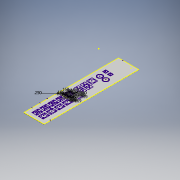
# Autodesk Inventor part: Box Connector Panel
Saved by Autodesk Inventor 2017 (Build 210142000, 142)
## iProperties
Created: 2017-03-01
Part Number: Box Connector Panel
Material: Generic
Document SubType Name: Modeling
Designer: slukej
Density: 1 g/cm^3
Appearance: Default
Author: slukej
Autodesk Inventor part; units mm, degrees
ref_plane "YZ Plane" through (0, 0, 0) normal (1, 0, 0) x (0, 1, 0)
ref_plane "XZ Plane" through (0, 0, 0) normal (0, 1, 0) x (-1, 0, 0)
ref_plane "XY Plane" through (0, 0, 0) normal (0, 0, 1) x (1, 0, 0)
sketch "Connector Plate" plane through (0, 0, 0) normal (0, 1, 0) x (-1, 0, 0)
  line L0 (-113.7687, 596.4285) -> (-243.9437, 596.4285)
  line L1 (-243.9437, 596.4285) -> (-243.9437, -13.1715)
  line L2 (-243.9437, -13.1715) -> (-113.7687, -13.1715)
  line L3 (-113.7687, -13.1715) -> (-113.7687, 596.4285)
  point P0 (0, 0)
  dimension "d0" = 130.175
  dimension "d1" = 609.6
  constraints: 8 end point, 2 parallel, 1 horizontal, 1 perpendicular
  measures "d0" distance of L2.end L1.end
  measures "d1" distance of L0.end L1.end
extrude "Extrusion1" add sketch "Connector Plate" along normal blind 3.175
sketch "DT04-2P - Exterior Panel (LS)" plane through (0, 3.175, 0) normal (0, 1, 0) x (1, 0, 0)
  line L0 (150.9797, -559.9795) -> (159.1077, -559.9795)
  line L1 (164.1877, -554.8995) -> (164.1877, -546.6445)
  line L2 (159.1077, -541.5645) -> (150.9797, -541.5645)
  line L3 (145.8997, -546.6445) -> (145.8997, -554.8995)
  circle A0 centre (143.8169, -565.9485) radius 2.159
  arc A1 (145.8997, -554.8995) -> (150.9797, -559.9795) centre (150.9797, -554.8995) ccw
  arc A2 (159.1077, -559.9795) -> (164.1877, -554.8995) centre (159.1077, -554.8995) ccw
  arc A3 (150.9797, -541.5645) -> (145.8997, -546.6445) centre (150.9797, -546.6445) ccw
  arc A4 (164.1877, -546.6445) -> (159.1077, -541.5645) centre (159.1077, -546.6445) ccw
  circle A5 centre (166.2705, -565.9485) radius 2.159
  circle A6 centre (143.8169, -535.5955) radius 2.159
  circle A7 centre (166.2705, -535.5955) radius 2.159
  line L4 (139.1687, -571.0285) -> (170.9187, -571.0285)
  line L5 (170.9187, -571.0285) -> (170.9187, -530.5155)
  line L6 (170.9187, -530.5155) -> (139.1687, -530.5155)
  line L7 (139.1687, -530.5155) -> (139.1687, -571.0285)
  line L8 (113.7687, -596.4285) -> (243.9437, -596.4285) projected
  line L9 (243.9437, -596.4285) -> (243.9437, 13.1715) projected
  line L10 (243.9437, 13.1715) -> (113.7687, 13.1715) projected
  line L11 (113.7687, 13.1715) -> (113.7687, -596.4285) projected
  line L12 (113.7687, 13.1715) -> (113.7687, -596.4285) projected
  line L13 (113.7687, -596.4285) -> (243.9437, -596.4285) projected
  line L14 (243.9437, 13.1715) -> (113.7687, 13.1715) projected
  arc A8 (150.9797, -490.7645) -> (145.8997, -495.8445) centre (150.9797, -495.8445) ccw
  line L15 (159.1077, -490.7645) -> (150.9797, -490.7645)
  arc A9 (164.1877, -495.8445) -> (159.1077, -490.7645) centre (159.1077, -495.8445) ccw
  arc A10 (145.8997, -504.0995) -> (150.9797, -509.1795) centre (150.9797, -504.0995) ccw
  line L16 (139.1687, -479.7155) -> (139.1687, -520.2285)
  arc A11 (159.1077, -509.1795) -> (164.1877, -504.0995) centre (159.1077, -504.0995) ccw
  line L17 (170.9187, -520.2285) -> (170.9187, -479.7155)
  line L18 (170.9187, -479.7155) -> (139.1687, -479.7155)
  circle A12 centre (166.2705, -484.7955) radius 2.159
  circle A13 centre (166.2705, -515.1485) radius 2.159
  line L19 (150.9797, -509.1795) -> (159.1077, -509.1795)
  circle A14 centre (143.8169, -515.1485) radius 2.159
  line L20 (164.1877, -504.0995) -> (164.1877, -495.8445)
  line L21 (145.8997, -495.8445) -> (145.8997, -504.0995)
  circle A15 centre (143.8169, -484.7955) radius 2.159
  line L22 (139.1687, -520.2285) -> (170.9187, -520.2285)
  arc A16 (150.9797, -439.9645) -> (145.8997, -445.0445) centre (150.9797, -445.0445) ccw
  line L23 (159.1077, -439.9645) -> (150.9797, -439.9645)
  arc A17 (164.1877, -445.0445) -> (159.1077, -439.9645) centre (159.1077, -445.0445) ccw
  arc A18 (145.8997, -453.2995) -> (150.9797, -458.3795) centre (150.9797, -453.2995) ccw
  line L24 (139.1687, -428.9155) -> (139.1687, -469.4285)
  arc A19 (159.1077, -458.3795) -> (164.1877, -453.2995) centre (159.1077, -453.2995) ccw
  line L25 (170.9187, -469.4285) -> (170.9187, -428.9155)
  line L26 (170.9187, -428.9155) -> (139.1687, -428.9155)
  circle A20 centre (166.2705, -433.9955) radius 2.159
  circle A21 centre (166.2705, -464.3485) radius 2.159
  line L27 (150.9797, -458.3795) -> (159.1077, -458.3795)
  circle A22 centre (143.8169, -464.3485) radius 2.159
  line L28 (164.1877, -453.2995) -> (164.1877, -445.0445)
  line L29 (145.8997, -445.0445) -> (145.8997, -453.2995)
  circle A23 centre (143.8169, -433.9955) radius 2.159
  line L30 (139.1687, -469.4285) -> (170.9187, -469.4285)
  arc A24 (150.9797, -389.1645) -> (145.8997, -394.2445) centre (150.9797, -394.2445) ccw
  line L31 (159.1077, -389.1645) -> (150.9797, -389.1645)
  arc A25 (164.1877, -394.2445) -> (159.1077, -389.1645) centre (159.1077, -394.2445) ccw
  arc A26 (145.8997, -402.4995) -> (150.9797, -407.5795) centre (150.9797, -402.4995) ccw
  line L32 (139.1687, -378.1155) -> (139.1687, -418.6285)
  arc A27 (159.1077, -407.5795) -> (164.1877, -402.4995) centre (159.1077, -402.4995) ccw
  line L33 (170.9187, -418.6285) -> (170.9187, -378.1155)
  line L34 (170.9187, -378.1155) -> (139.1687, -378.1155)
  circle A28 centre (166.2705, -383.1955) radius 2.159
  circle A29 centre (166.2705, -413.5485) radius 2.159
  line L35 (150.9797, -407.5795) -> (159.1077, -407.5795)
  circle A30 centre (143.8169, -413.5485) radius 2.159
  line L36 (164.1877, -402.4995) -> (164.1877, -394.2445)
  line L37 (145.8997, -394.2445) -> (145.8997, -402.4995)
  circle A31 centre (143.8169, -383.1955) radius 2.159
  line L38 (139.1687, -418.6285) -> (170.9187, -418.6285)
  point P0 (0, 0)
  point P1 (145.8997, -559.9795)
  point P2 (164.1877, -541.5645)
  point P3 (145.8997, -541.5645)
  point P4 (145.8997, -490.7645)
  point P5 (164.1877, -490.7645)
  point P6 (145.8997, -509.1795)
  point P7 (113.7687, -545.6285)
  point P8 (145.8997, -439.9645)
  point P9 (164.1877, -439.9645)
  point P10 (145.8997, -458.3795)
  point P11 (113.7687, -494.8285)
  point P12 (145.8997, -389.1645)
  point P13 (164.1877, -389.1645)
  point P14 (145.8997, -407.5795)
  point P15 (113.7687, -444.0285)
  dimension "d166" = 18.288
  dimension "d167" = 18.415
  dimension "d168" = 4.318
  dimension "d169" = 5.08
  dimension "d170" = 5.08
  dimension "d171" = 5.08
  dimension "d172" = 5.08
  dimension "d173" = 4.318
  dimension "d174" = 4.318
  dimension "d175" = 4.318
  dimension "d176" = 5.969
  dimension "d177" = 22.4536
  dimension "d178" = 0
  dimension "d179" = 2.0828
  dimension "d180" = 30.353
  dimension "d181" = 0
  dimension "d182" = 22.4536
  dimension "d183" = 5.969
  dimension "d184" = 31.75
  dimension "d185" = 40.513
  dimension "d186" = 5.08
  dimension "d187" = 4.6482
  dimension "d272" = 25.4
  dimension "d273" = 25.4
  dimension "d351" = 50.8
  constraints: 64 end point, 32 centre point, 32 point on circle, 24 point on line, 8 tangent, 4 parallel, 2 horizontal, 2 perpendicular, 1 vertical, 120 other
  measures "d166" distance of point (164.188, -541.564) point (145.9, -541.564)
  measures "d167" distance of point (145.9, -541.564) point (145.9, -559.979)
  measures "d168" diameter of A0
  measures "d169" radius of A1
  measures "d170" radius of A2
  measures "d171" radius of A3
  measures "d172" radius of A4
  measures "d173" diameter of A5
  measures "d174" diameter of A6
  measures "d175" diameter of A7
  measures "d176" distance from line of A6.centre L2
  measures "d177" distance of A7.centre A6.centre
  measures "d178" vertical distance of A6.centre A7.centre
  measures "d179" distance from line of L3 A6.centre
  measures "d180" distance of A6.centre A0.centre
  measures "d181" horizontal distance of A6.centre A0.centre
  measures "d182" distance of A0.centre A5.centre
  measures "d183" distance from line of L0 A5.centre
  measures "d184" distance of L5.end L6.end
  measures "d185" distance of L4.end L5.end
  measures "d186" distance from line of L6 A6.centre
  measures "d187" distance from line of L7 A6.centre
  measures "d272" distance between parallel lines of L12 L7
  measures "d273" distance between parallel lines of L13 L4
  measures "d351" distance of L2.start L15.start
sketch "DT04-3P - VSCADA I/O" plane through (0, 3.175, 0) normal (0, 1, 0) x (1, 0, 0)
  circle A0 centre (196.9537, -550.772) radius 12.7
  circle A1 centre (185.7269, -565.9485) radius 2.159
  circle A2 centre (185.7269, -535.5955) radius 2.159
  circle A3 centre (208.1805, -565.9485) radius 2.159
  circle A4 centre (208.1805, -535.5955) radius 2.159
  line L0 (181.0787, -571.0285) -> (212.8287, -571.0285)
  line L1 (212.8287, -571.0285) -> (212.8287, -530.5155)
  line L2 (212.8287, -530.5155) -> (181.0787, -530.5155)
  line L3 (181.0787, -530.5155) -> (181.0787, -571.0285)
  line L4 (113.7687, 13.1715) -> (113.7687, -596.4285) projected
  line L5 (113.7687, -596.4285) -> (243.9437, -596.4285) projected
  line L6 (243.9437, 13.1715) -> (113.7687, 13.1715) projected
  line L7 (243.9437, -596.4285) -> (243.9437, 13.1715) projected
  line L8 (170.9187, -530.5155) -> (139.1687, -530.5155) projected
  line L9 (170.9187, -571.0285) -> (170.9187, -530.5155) projected
  circle A5 centre (196.9537, -499.972) radius 12.7
  circle A6 centre (185.7269, -484.7955) radius 2.159
  line L10 (181.0787, -479.7155) -> (181.0787, -520.2285)
  line L11 (212.8287, -479.7155) -> (181.0787, -479.7155)
  line L12 (212.8287, -520.2285) -> (212.8287, -479.7155)
  circle A7 centre (185.7269, -515.1485) radius 2.159
  line L13 (181.0787, -520.2285) -> (212.8287, -520.2285)
  circle A8 centre (208.1805, -515.1485) radius 2.159
  circle A9 centre (208.1805, -484.7955) radius 2.159
  circle A10 centre (196.9537, -449.172) radius 12.7
  circle A11 centre (185.7269, -433.9955) radius 2.159
  line L14 (181.0787, -428.9155) -> (181.0787, -469.4285)
  line L15 (212.8287, -428.9155) -> (181.0787, -428.9155)
  line L16 (212.8287, -469.4285) -> (212.8287, -428.9155)
  circle A12 centre (185.7269, -464.3485) radius 2.159
  line L17 (181.0787, -469.4285) -> (212.8287, -469.4285)
  circle A13 centre (208.1805, -464.3485) radius 2.159
  circle A14 centre (208.1805, -433.9955) radius 2.159
  circle A15 centre (196.9537, -398.372) radius 12.7
  circle A16 centre (185.7269, -383.1955) radius 2.159
  line L18 (181.0787, -378.1155) -> (181.0787, -418.6285)
  line L19 (212.8287, -378.1155) -> (181.0787, -378.1155)
  line L20 (212.8287, -418.6285) -> (212.8287, -378.1155)
  circle A17 centre (185.7269, -413.5485) radius 2.159
  line L21 (181.0787, -418.6285) -> (212.8287, -418.6285)
  circle A18 centre (208.1805, -413.5485) radius 2.159
  circle A19 centre (208.1805, -383.1955) radius 2.159
  point P0 (0, 0)
  point P1 (170.9187, -479.7155)
  point P2 (170.9187, -520.2285)
  point P3 (170.9187, -428.9155)
  point P4 (170.9187, -469.4285)
  point P5 (170.9187, -378.1155)
  point P6 (170.9187, -418.6285)
  dimension "d217" = 25.4
  dimension "d218" = 4.318
  dimension "d219" = 4.318
  dimension "d220" = 4.318
  dimension "d221" = 4.318
  dimension "d222" = 11.2268
  dimension "d223" = 11.2268
  dimension "d224" = 11.2268
  dimension "d225" = 11.2268
  dimension "d226" = 15.1765
  dimension "d227" = 15.1765
  dimension "d228" = 15.1765
  dimension "d229" = 15.1765
  dimension "d230" = 31.75
  dimension "d231" = 40.513
  dimension "d232" = 5.08
  dimension "d233" = 4.6482
  dimension "d343" = 10.16
  dimension "d344" = 25.4
  dimension "d358" = 50.8
  constraints: 32 end point, 20 centre point, 2 parallel, 1 horizontal, 1 perpendicular, 1 vertical, 60 other
  measures "d217" diameter of A0
  measures "d218" diameter of A1
  measures "d219" diameter of A2
  measures "d220" diameter of A3
  measures "d221" diameter of A4
  measures "d222" horizontal distance of A0.centre A2.centre
  measures "d223" horizontal distance of A0.centre A1.centre
  measures "d224" horizontal distance of A0.centre A3.centre
  measures "d225" horizontal distance of A0.centre A4.centre
  measures "d226" vertical distance of A0.centre A2.centre
  measures "d227" vertical distance of A1.centre A0.centre
  measures "d228" vertical distance of A0.centre A3.centre
  measures "d229" vertical distance of A0.centre A4.centre
  measures "d230" distance of L1.end L2.end
  measures "d231" distance of L1.end L0.end
  measures "d232" distance from line of A2.centre L2
  measures "d233" distance from line of L3 A2.centre
  measures "d343" distance between parallel lines of L9 L3
  measures "d344" distance between parallel lines of L5 L0
  measures "d358" distance of A2.centre A6.centre
sketch "DT04-4P - Safety Loop" plane through (0, 3.175, 0) normal (0, 1, 0) x (1, 0, 0)
  line L0 (151.1575, -358.748) -> (159.4379, -358.748)
  line L1 (165.7879, -352.398) -> (165.7879, -343)
  line L2 (159.4379, -336.65) -> (151.1575, -336.65)
  line L3 (144.8075, -343) -> (144.8075, -352.398)
  arc A0 (144.8075, -352.398) -> (151.1575, -358.748) centre (151.1575, -352.398) ccw
  arc A1 (151.1575, -336.65) -> (144.8075, -343) centre (151.1575, -343) ccw
  arc A2 (165.7879, -343) -> (159.4379, -336.65) centre (159.4379, -343) ccw
  arc A3 (159.4379, -358.748) -> (165.7879, -352.398) centre (159.4379, -352.398) ccw
  circle A4 centre (143.8169, -362.8755) radius 2.1463
  circle A5 centre (166.5245, -332.5225) radius 2.1463
  circle A6 centre (166.5245, -362.8755) radius 2.1463
  circle A7 centre (144.0709, -332.5225) radius 2.1463
  line L4 (139.1687, -367.9555) -> (170.9187, -367.9555)
  line L5 (170.9187, -367.9555) -> (170.9187, -327.4425)
  line L6 (170.9187, -327.4425) -> (139.1687, -327.4425)
  line L7 (139.1687, -327.4425) -> (139.1687, -367.9555)
  line L8 (113.7687, 13.1715) -> (113.7687, -596.4285) projected
  line L9 (113.7687, -596.4285) -> (243.9437, -596.4285) projected
  line L10 (212.8287, -469.4285) -> (212.8287, -428.9155) projected
  line L11 (170.9187, -378.1155) -> (139.1687, -378.1155) projected
  point P0 (0, 0)
  point P1 (165.7879, -336.65)
  point P2 (165.7879, -358.748)
  point P3 (144.8075, -336.65)
  dimension "d76" = 20.9804
  dimension "d77" = 22.098
  dimension "d78" = 6.35
  dimension "d79" = 4.2926
  dimension "d80" = 4.2926
  dimension "d81" = 4.2926
  dimension "d82" = 4.2926
  dimension "d83" = 0.9906
  dimension "d84" = 0.7366
  dimension "d85" = 0.7366
  dimension "d86" = 0.7366
  dimension "d87" = 4.1275
  dimension "d88" = 4.1275
  dimension "d89" = 4.1275
  dimension "d90" = 4.1275
  dimension "d188" = 31.75
  dimension "d189" = 40.513
  dimension "d190" = 5.08
  dimension "d191" = 4.6482
  dimension "d397" = 10.16
  dimension "d398" = 25.4
  constraints: 16 end point, 8 centre point, 8 point on circle, 8 tangent, 6 point on line, 4 parallel, 3 equal radius, 2 horizontal, 2 perpendicular
  measures "d76" distance of point (144.807, -336.65) point (165.788, -336.65)
  measures "d77" distance of point (165.788, -336.65) point (165.788, -358.748)
  measures "d78" radius of A0
  measures "d79" diameter of A4
  measures "d80" diameter of A5
  measures "d81" diameter of A6
  measures "d82" diameter of A7
  measures "d83" distance from line of L3 A4.centre
  measures "d84" distance from line of L1 A6.centre
  measures "d85" distance from line of L1 A5.centre
  measures "d86" distance from line of A7.centre L3
  measures "d87" distance from line of L0 A4.centre
  measures "d88" distance from line of L0 A6.centre
  measures "d89" distance from line of L2 A5.centre
  measures "d90" distance from line of L2 A7.centre
  measures "d188" distance of L6.end L5.end
  measures "d189" distance of L5.end L4.end
  measures "d190" distance from line of A7.centre L6
  measures "d191" distance from line of L7 A4.centre
  measures "d397" distance between parallel lines of L11 L4
  measures "d398" distance between parallel lines of L8 L7
sketch "DT04-6P - Exterior Panel (RS)" plane through (0, 3.175, 0) normal (0, 1, 0) x (1, 0, 0)
  line L0 (160.6825, -297.5975) -> (173.4079, -297.5975)
  line L1 (179.7579, -291.2475) -> (179.7579, -281.8495)
  line L2 (173.4079, -275.4995) -> (160.6825, -275.4995)
  line L3 (154.3325, -281.8495) -> (154.3325, -291.2475)
  arc A0 (154.3325, -291.2475) -> (160.6825, -297.5975) centre (160.6825, -291.2475) ccw
  arc A1 (173.4079, -297.5975) -> (179.7579, -291.2475) centre (173.4079, -291.2475) ccw
  arc A2 (179.7579, -281.8495) -> (173.4079, -275.4995) centre (173.4079, -281.8495) ccw
  arc A3 (160.6825, -275.4995) -> (154.3325, -281.8495) centre (160.6825, -281.8495) ccw
  circle A4 centre (147.7412, -286.5485) radius 2.8067
  circle A5 centre (186.3492, -286.5485) radius 3.175
  line L4 (139.1687, -302.0425) -> (193.9057, -302.0425)
  line L5 (193.9057, -302.0425) -> (193.9057, -271.0545)
  line L6 (193.9057, -271.0545) -> (139.1687, -271.0545)
  line L7 (139.1687, -271.0545) -> (139.1687, -302.0425)
  line L8 (113.7687, 13.1715) -> (113.7687, -596.4285) projected
  line L9 (113.7687, -596.4285) -> (243.9437, -596.4285) projected
  line L10 (212.8287, -530.5155) -> (181.0787, -530.5155) projected
  line L11 (212.8287, -571.0285) -> (212.8287, -530.5155) projected
  line L12 (160.6825, -256.4495) -> (173.4079, -256.4495)
  line L13 (179.7579, -250.0995) -> (179.7579, -240.7015)
  line L14 (173.4079, -234.3515) -> (160.6825, -234.3515)
  line L15 (154.3325, -240.7015) -> (154.3325, -250.0995)
  arc A6 (154.3325, -250.0995) -> (160.6825, -256.4495) centre (160.6825, -250.0995) ccw
  line L16 (139.1687, -229.9065) -> (139.1687, -260.8945)
  circle A7 centre (147.7412, -245.4005) radius 2.8067
  arc A8 (160.6825, -234.3515) -> (154.3325, -240.7015) centre (160.6825, -240.7015) ccw
  arc A9 (173.4079, -256.4495) -> (179.7579, -250.0995) centre (173.4079, -250.0995) ccw
  arc A10 (179.7579, -240.7015) -> (173.4079, -234.3515) centre (173.4079, -240.7015) ccw
  line L17 (193.9057, -229.9065) -> (139.1687, -229.9065)
  line L18 (139.1687, -260.8945) -> (193.9057, -260.8945)
  circle A11 centre (186.3492, -245.4005) radius 3.175
  line L19 (193.9057, -260.8945) -> (193.9057, -229.9065)
  line L20 (139.1687, -367.9555) -> (170.9187, -367.9555) projected
  line L21 (170.9187, -327.4425) -> (139.1687, -327.4425) projected
  line L22 (170.9187, -367.9555) -> (170.9187, -327.4425) projected
  line L23 (139.1687, -327.4425) -> (139.1687, -367.9555) projected
  point P0 (0, 0)
  point P1 (212.8287, -529.8805)
  point P2 (212.8287, -489.3675)
  point P3 (181.0787, -489.3675)
  point P4 (243.9437, -555.2805)
  dimension "d268" = 6.35
  dimension "d269" = 25.4254
  dimension "d270" = 22.098
  dimension "d271" = 5.6134
  dimension "d290" = 6.35
  dimension "d291" = 6.5913
  dimension "d292" = 6.5913
  dimension "d293" = 11.049
  dimension "d294" = 11.049
  dimension "d295" = 54.737
  dimension "d296" = 30.988
  dimension "d297" = 15.494
  dimension "d298" = 14.1478
  dimension "d365" = 41.148
  dimension "d401" = 25.4
  dimension "d402" = 0
  constraints: 32 end point, 16 point on circle, 12 centre point, 8 tangent, 4 parallel, 3 equal radius, 2 horizontal, 2 perpendicular, 1 vertical, 36 other
  measures "d268" radius of A0
  measures "d269" distance between parallel lines of L1 L3
  measures "d270" distance between parallel lines of L2 L0
  measures "d271" diameter of A4
  measures "d290" diameter of A5
  measures "d291" distance from line of A4.centre L3
  measures "d292" distance from line of A5.centre L1
  measures "d293" distance from line of A4.centre L2
  measures "d294" distance from line of L2 A5.centre
  measures "d295" distance of L6.end L5.end
  measures "d296" distance of L5.end L4.end
  measures "d297" distance from line of A4.centre L6
  measures "d298" distance between parallel lines of L1 L5
  measures "d365" distance of L0.start L12.start
  measures "d401" distance between parallel lines of L21 L4
  measures "d402" distance between parallel lines of L23 L7
sketch "DT04-6P - Exterior Panel (RS) ALT" plane through (0, 3.175, 0) normal (0, 1, 0) x (1, 0, 0)
  line L0 (48.3979, -171.3115) -> (61.0979, -171.3115)
  line L1 (67.4479, -164.9615) -> (67.4479, -152.2615)
  line L2 (61.0979, -145.9115) -> (48.3979, -145.9115)
  line L3 (42.0479, -152.2615) -> (42.0479, -164.9615)
  arc A0 (42.0479, -164.9615) -> (48.3979, -171.3115) centre (48.3979, -164.9615) ccw
  arc A1 (61.0979, -171.3115) -> (67.4479, -164.9615) centre (61.0979, -164.9615) ccw
  arc A2 (67.4479, -152.2615) -> (61.0979, -145.9115) centre (61.0979, -152.2615) ccw
  arc A3 (48.3979, -145.9115) -> (42.0479, -152.2615) centre (48.3979, -152.2615) ccw
  circle A4 centre (42.7464, -181.1159) radius 2.159
  circle A5 centre (66.7494, -136.1071) radius 2.159
  circle A6 centre (66.7494, -181.1159) radius 2.159
  circle A7 centre (42.7464, -136.1071) radius 2.159
  line L4 (36.9933, -186.107) -> (72.5025, -186.107)
  line L5 (72.5025, -186.107) -> (72.5025, -131.116)
  line L6 (72.5025, -131.116) -> (36.9933, -131.116)
  line L7 (36.9933, -131.116) -> (36.9933, -186.107)
  point P0 (0, 0)
  point P1 (67.4479, -145.9115)
  point P2 (67.4479, -171.3115)
  point P3 (42.0479, -145.9115)
  dimension "d91" = 25.4
  dimension "d92" = 25.4
  dimension "d93" = 6.35
  dimension "d94" = 4.318
  dimension "d95" = 4.318
  dimension "d96" = 4.318
  dimension "d97" = 4.318
  dimension "d98" = 9.8044
  dimension "d99" = 9.8044
  dimension "d100" = 9.8044
  dimension "d101" = 9.8044
  dimension "d102" = 0.6985
  dimension "d103" = 24.003
  dimension "d104" = 0.6985
  dimension "d105" = 24.003
  dimension "d192" = 35.5092
  dimension "d193" = 54.991
  dimension "d194" = 5.7531
  dimension "d195" = 4.9911
  constraints: 16 end point, 8 centre point, 8 point on circle, 8 tangent, 6 point on line, 4 parallel, 3 equal radius, 2 horizontal, 2 perpendicular
  measures "d91" distance of point (42.048, -145.911) point (67.448, -145.911)
  measures "d92" distance of point (67.448, -145.911) point (67.448, -171.311)
  measures "d93" radius of A0
  measures "d94" diameter of A4
  measures "d95" diameter of A5
  measures "d96" diameter of A6
  measures "d97" diameter of A7
  measures "d98" distance from line of L0 A4.centre
  measures "d99" distance from line of L0 A6.centre
  measures "d100" distance from line of L2 A5.centre
  measures "d101" distance from line of L2 A7.centre
  measures "d102" distance from line of L3 A4.centre
  measures "d103" distance of A6.centre A4.centre
  measures "d104" distance from line of L3 A7.centre
  measures "d105" distance of A7.centre A5.centre
  measures "d192" distance of L6.end L5.end
  measures "d193" distance of L5.end L4.end
  measures "d194" distance from line of A7.centre L7
  measures "d195" distance from line of A5.centre L6
sketch "DT04-12P - Interior Panel" plane through (0, 3.175, 0) normal (0, 1, 0) x (1, 0, 0)
  line L0 (193.4485, -319.4796) -> (204.2689, -319.4796)
  line L1 (210.6189, -325.8296) -> (210.6189, -354.9634)
  line L2 (204.2689, -361.3134) -> (193.4485, -361.3134)
  line L3 (187.0985, -354.9634) -> (187.0985, -325.8296)
  arc A0 (187.0985, -354.9634) -> (193.4485, -361.3134) centre (193.4485, -354.9634) ccw
  arc A1 (204.2689, -361.3134) -> (210.6189, -354.9634) centre (204.2689, -354.9634) ccw
  arc A2 (210.6189, -325.8296) -> (204.2689, -319.4796) centre (204.2689, -325.8296) ccw
  arc A3 (193.4485, -319.4796) -> (187.0985, -325.8296) centre (193.4485, -325.8296) ccw
  circle A4 centre (186.9207, -317.9175) radius 2.1463
  circle A5 centre (210.7967, -317.9175) radius 2.1463
  circle A6 centre (210.7967, -362.8755) radius 2.1463
  circle A7 centre (186.9207, -362.8755) radius 2.1463
  line L4 (181.0787, -367.9555) -> (216.6387, -367.9555)
  line L5 (216.6387, -367.9555) -> (216.6387, -312.8375)
  line L6 (216.6387, -312.8375) -> (181.0787, -312.8375)
  line L7 (181.0787, -312.8375) -> (181.0787, -367.9555)
  line L8 (113.7687, 13.1715) -> (113.7687, -596.4285) projected
  line L9 (113.7687, -596.4285) -> (243.9437, -596.4285) projected
  line L10 (170.9187, -327.4425) -> (139.1687, -327.4425) projected
  line L11 (212.8287, -469.4285) -> (212.8287, -428.9155) projected
  line L12 (181.0787, -378.1155) -> (181.0787, -418.6285) projected
  line L13 (212.8287, -378.1155) -> (181.0787, -378.1155) projected
  point P0 (0, 0)
  point P1 (187.0985, -319.4796)
  point P2 (210.6189, -361.3134)
  point P3 (187.0985, -361.3134)
  dimension "d106" = 23.5204
  dimension "d107" = 41.8338
  dimension "d108" = 6.35
  dimension "d110" = 0.1778
  dimension "d111" = 23.876
  dimension "d112" = 0.1778
  dimension "d113" = 1.5621
  dimension "d114" = 23.876
  dimension "d115" = 1.5621
  dimension "d116" = 1.5621
  dimension "d117" = 1.5621
  dimension "d196" = 35.56
  dimension "d197" = 55.118
  dimension "d198" = 5.08
  dimension "d199" = 5.842
  dimension "d305" = 4.2926
  dimension "d306" = 4.2926
  dimension "d307" = 4.2926
  dimension "d308" = 4.2926
  dimension "d399" = 0
  dimension "d400" = 10.16
  constraints: 16 end point, 8 centre point, 8 point on circle, 8 tangent, 6 point on line, 4 parallel, 3 equal radius, 2 horizontal, 2 perpendicular
  measures "d106" distance of point (210.619, -361.313) point (187.098, -361.313)
  measures "d107" distance of point (187.098, -319.48) point (187.098, -361.313)
  measures "d108" radius of A0
  measures "d110" distance from line of L3 A4.centre
  measures "d111" distance of A4.centre A5.centre
  measures "d112" distance from line of L3 A7.centre
  measures "d113" distance from line of A4.centre L0
  measures "d114" distance of A6.centre A7.centre
  measures "d115" distance from line of L0 A5.centre
  measures "d116" distance from line of L2 A7.centre
  measures "d117" distance from line of L2 A6.centre
  measures "d196" distance of L6.end L5.end
  measures "d197" distance of L6.end L4.start
  measures "d198" distance from line of A4.centre L6
  measures "d199" distance from line of L7 A4.centre
  measures "d305" diameter of A4
  measures "d306" diameter of A5
  measures "d307" diameter of A6
  measures "d308" diameter of A7
  measures "d399" distance between parallel lines of L12 L7
  measures "d400" distance between parallel lines of L13 L4
sketch "USB/Ethernet Mounts" plane through (0, 3.175, 0) normal (0, 1, 0) x (1, 0, 0)
  arc A0 (168.9187, -143.2107) -> (168.9187, -155.8202) centre (156.4187, -149.5155) ccw
  line L0 (168.9187, -155.8202) -> (168.9187, -143.2107)
  circle A1 centre (156.4187, -149.5155) radius 17.25
  line L1 (113.7687, -596.4285) -> (243.9437, -596.4285) projected
  line L2 (243.9437, -596.4285) -> (243.9437, 13.1715) projected
  line L3 (243.9437, 13.1715) -> (113.7687, 13.1715) projected
  line L4 (113.7687, 13.1715) -> (113.7687, -596.4285) projected
  line L5 (113.7687, -596.4285) -> (243.9437, -596.4285) projected
  line L6 (170.9187, -378.1155) -> (139.1687, -378.1155) projected
  arc A2 (207.0187, -143.2107) -> (207.0187, -155.8202) centre (194.5187, -149.5155) ccw
  line L7 (207.0187, -155.8202) -> (207.0187, -143.2107)
  circle A3 centre (194.5187, -149.5155) radius 17.25
  point P0 (0, 0)
  dimension "d310" = 12.5
  dimension "d312" = 26.5
  dimension "d313" = 34.5
  dimension "d316" = 3.25
  dimension "d372" = 228.6
  dimension "d375" = 38.1
  dimension "d385" = 42.65
  constraints: 4 centre point, 4 end point, 4 point on circle, 2 coincident, 1 horizontal, 1 vertical, 7 other
  measures "d310" distance from line of L0 A0.centre
  measures "d313" diameter of A1
  measures "d316" radial gap between concentric circles of A1 A0
  measures "d372" distance from line of A0.centre L6
  measures "d375" distance of A0.centre A2.centre
  measures "d385" distance from line of L4 A0.centre
sketch "HDMI Mount" plane through (0, 3.175, 0) normal (0, 1, 0) x (1, 0, 0)
  line L0 (175.7447, -219.7465) -> (139.1687, -219.7465)
  line L1 (139.1687, -219.7465) -> (139.1687, -183.1705)
  line L2 (139.1687, -183.1705) -> (175.7447, -183.1705)
  line L3 (175.7447, -183.1705) -> (175.7447, -219.7465)
  line L4 (113.7687, 13.1715) -> (113.7687, -596.4285) projected
  circle A0 centre (157.4567, -201.4585) radius 15.113
  line L5 (216.6387, -312.8375) -> (181.0787, -312.8375) projected
  line L6 (193.9057, -229.9065) -> (139.1687, -229.9065) projected
  point P0 (0, 0)
  point P1 (214.17, -4.8669)
  point P2 (194.5187, -149.5155)
  dimension "d336" = 36.576
  dimension "d337" = 36.576
  dimension "d340" = 30.226
  dimension "d341" = 18.288
  dimension "d342" = 18.288
  dimension "d403" = 10.16
  dimension "d404" = 25.4
  constraints: 8 end point, 2 parallel, 1 centre point, 1 horizontal, 1 perpendicular
  measures "d336" distance of L1.end L2.end
  measures "d337" distance of L2.end L0.start
  measures "d340" diameter of A0
  measures "d341" distance from line of L1 A0.centre
  measures "d342" distance from line of L2 A0.centre
  measures "d403" distance between parallel lines of L6 L0
  measures "d404" distance between parallel lines of L4 L1
sketch "CircuitB Breakers" plane through (0, 3.175, 0) normal (0, 1, 0) x (1, 0, 0)
  line L0 (139.1687, -114.5075) -> (158.4727, -114.5075)
  line L1 (158.4727, -114.5075) -> (158.4727, -95.2035)
  line L2 (158.4727, -95.2035) -> (139.1687, -95.2035)
  line L3 (139.1687, -95.2035) -> (139.1687, -114.5075)
  circle A0 centre (148.8207, -104.8555) radius 8.001
  line L4 (113.7687, 13.1715) -> (113.7687, -596.4285) projected
  circle A1 centre (156.4187, -149.5155) radius 17.25 projected
  line L5 (169.6487, -114.5075) -> (188.9527, -114.5075)
  line L6 (188.9527, -114.5075) -> (188.9527, -95.2035)
  line L7 (188.9527, -95.2035) -> (169.6487, -95.2035)
  line L8 (169.6487, -95.2035) -> (169.6487, -114.5075)
  circle A2 centre (179.3007, -104.8555) radius 8.001
  point P0 (0, 0)
  point P1 (144.2487, 13.1715)
  dimension "d380" = 19.304
  dimension "d381" = 19.304
  dimension "d382" = 16.002
  dimension "d383" = 9.652
  dimension "d384" = 9.652
  dimension "d388" = 25.4
  dimension "d389" = 44.66
  dimension "d392" = 30.48
  dimension "d405" = 34.5
  constraints: 16 end point, 2 centre point, 2 horizontal, 2 parallel, 1 collinear, 1 perpendicular, 10 other
  measures "d380" distance of L2.end L1.end
  measures "d381" distance of L1.end L0.end
  measures "d382" diameter of A0
  measures "d383" distance from line of L2 A0.centre
  measures "d384" distance from line of L1 A0.centre
  measures "d388" distance between parallel lines of L4 L3
  measures "d389" vertical distance of A0.centre A1.centre
  measures "d392" distance of L0.start L5.start
  measures "d405" diameter of A1
body "Solid1"
